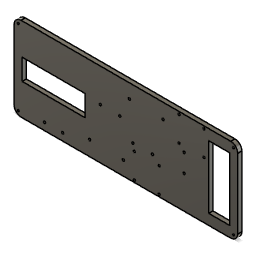
Base_Robot_Sanchez v22 (Autodesk Fusion 360 design; units mm, degrees)
Autodesk Fusion 360 part; units mm, degrees
sketch "Esquisse1" plane through (0, 0, 0) normal (0, 0, 1) x (1, 0, 0)
  circle A0 centre (114, 54) radius 1.41
  circle A1 centre (-194, -54) radius 1.41
  circle A2 centre (114, -54) radius 1.41
  circle A3 centre (-194, 54) radius 1.41
  line L0 (108.5, 45.0007) -> (108.5, -44.9993)
  line L1 (108.5, 45.0007) -> (78.5, 45.0007)
  line L2 (78.5, 45.0007) -> (78.5, -44.9993)
  line L3 (78.5, -44.9993) -> (108.5, -44.9993)
  circle A4 centre (43.3, 13) radius 1.6
  circle A5 centre (43.3, -13) radius 1.6
  line L4 (-188.5, 15.01) -> (-188.5, -14.99)
  line L5 (-188.5, -14.99) -> (-98.5, -14.99)
  line L6 (-98.5, -14.99) -> (-98.5, 15.01)
  line L7 (-98.5, 15.01) -> (-188.5, 15.01)
  circle A6 centre (-156.5, -49.69) radius 1.6
  circle A7 centre (-130.5, -49.69) radius 1.6
  circle A8 centre (71.6331, 20.8253) radius 1.5
  circle A9 centre (71.6331, 56.3653) radius 1.5
  circle A10 centre (-27.9142, -21.394) radius 1.5
  circle A11 centre (7.6258, -56.934) radius 1.5
  circle A12 centre (-27.9142, -56.934) radius 1.5
  circle A13 centre (7.6258, -21.394) radius 1.5
  circle A14 centre (-43.6012, -39.9923) radius 1.5875
  circle A15 centre (-91.8612, -38.7223) radius 1.5875
  circle A16 centre (-48.6812, 12.0777) radius 1.5875
  circle A17 centre (-76.6212, 12.0777) radius 1.5875
  circle A18 centre (-30.0015, -12.1732) radius 1.5875
  circle A19 centre (-2.0615, -12.1732) radius 1.5875
  circle A20 centre (-35.0815, 39.8968) radius 1.5875
  line L8 (-190, 60) -> (110, 60)
  line L9 (120, 50) -> (120, -50)
  line L10 (110, -60) -> (-190, -60)
  line L11 (-200, -50) -> (-200, 50)
  arc A21 (-190, 60) -> (-200, 50) centre (-190, 50) ccw
  arc A22 (-200, -50) -> (-190, -60) centre (-190, -50) ccw
  arc A23 (110, -60) -> (120, -50) centre (110, -50) ccw
  arc A24 (120, 50) -> (110, 60) centre (110, 50) ccw
  circle A25 centre (13.1785, 38.6268) radius 1.5875
  circle A26 centre (36.0931, 56.3653) radius 1.5
  circle A27 centre (36.0931, 20.8253) radius 1.5
  point P0 (-6.5496, 0)
  point P1 (-6.5496, 0)
  point P2 (-140, 0)
  dimension "d56" = 30
  dimension "d57" = 90
  dimension "d59" = 3.2
  dimension "d60" = 30
  dimension "d64" = 30
  dimension "d65" = 3.2
  dimension "d115" = 3.2
  dimension "d117" = 3.2
  dimension "d134" = 10
  dimension "d135" = 10
  dimension "d136" = 10
  dimension "d137" = 10
  constraint coincident P1 P0
  constraint perpendicular L0 L1
  constraint perpendicular L1 L2
  constraint perpendicular L4 L5
  constraint perpendicular L5 L6
  constraint horizontal L8
  constraint vertical L9
  constraint horizontal L10
  constraint vertical L11
  constraint tangent L8 A21
  constraint tangent L11 A21
  constraint tangent L10 A22
  constraint tangent L11 A22
  constraint tangent L9 A23
  constraint tangent L10 A23
  constraint tangent L8 A24
  constraint tangent L9 A24
  measures "d56" distance of L0.start L1.end
  measures "d57" distance of L1.end L2.end
  measures "d59" diameter of A4
  measures "d60" distance of L4.start L4.end
  measures "d64" distance of L5.end L6.end
  measures "d65" diameter of A6
  measures "d115" diameter of A5
  measures "d117" diameter of A7
  measures "d134" radius of A21
  measures "d135" radius of A22
  measures "d136" radius of A23
  measures "d137" radius of A24
extrude "Extrusion1" add sketch "Esquisse1" along normal blind 6 contours L0 L1 L2 L3 | A4 | A5 | L4 L5 L6 L7 | A6 | A7 | A8 | A9 | A10 | A11 | A12 | A13 | A14 | A15 | A16 | A17 | A18 | A19 | A20 | L8 L9 L10 L11 A21 A22 A23 A24 | A25 | A26 | A27
extrude "Extrusion2" cut sketch "Esquisse1" along normal blind 6 contours L4 L5 L6 L7
extrude "Extrusion3" cut sketch "Esquisse1" along normal blind 6 contours L0 L1 L2 L3
extrude "Extrusion4" cut sketch "Esquisse1" along normal blind 6 contours A4 | A5
extrude "Extrusion5" cut sketch "Esquisse1" along normal blind 6 contours A6 | A7
extrude "Extrusion11" cut sketch "Esquisse1" along normal up to surface (6 mm away) contours A8 | A9 | A10 | A11 | A12 | A13 | A14 | A15 | A16 | A17 | A18 | A19 | A20
extrude "Extrusion12" cut sketch "Esquisse1" along normal up to surface (6 mm away) contours A25 | A26 | A27
